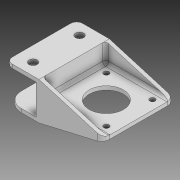
# Autodesk Inventor part: MotorBracket2
Saved by Autodesk Inventor 2020 (Build 240168000, 168)
## iProperties
Created: 2020-10-22
Part Number: MotorBracket2
Material: Generic
Document SubType Name: Modeling
Designer: DDeGo
Density: 1 g/cm^3
Appearance: Default
Author: DDeGo
Autodesk Inventor part; units mm, degrees
ref_plane "YZ Plane" through (0, 0, 0) normal (1, 0, 0) x (0, 1, 0)
ref_plane "XZ Plane" through (0, 0, 0) normal (0, 1, 0) x (-1, 0, 0)
ref_plane "XY Plane" through (0, 0, 0) normal (0, 0, 1) x (1, 0, 0)
sketch "Sketch1" plane through (0, 0, 0) normal (0, 0, 1) x (1, 0, 0)
  line L0 (0, 0) -> (20, 0)
  line L1 (20, 0) -> (20, 2.5) construction
  line L2 (20, 2.5) -> (0, 2.5)
  line L3 (0, 2.5) -> (0, 0)
  line L4 (0, 25.3) -> (20, 25.3)
  line L5 (20, 25.3) -> (20, 22.8) construction
  line L6 (20, 22.8) -> (0, 22.8)
  line L7 (0, 22.8) -> (0, 25.3)
  line L8 (20, 22.8) -> (20, 2.5)
  line L9 (20, 25.3) -> (22, 25.3)
  line L10 (22, 25.3) -> (65.3, 12.5) construction
  line L11 (65.3, 12.5) -> (65.3, 10)
  line L12 (65.3, 10) -> (22, 0) construction
  line L13 (22, 0) -> (20, 0)
  line L14 (22, 25.3) -> (22, 0) construction
  line L15 (22, 25.3) -> (22, 12.5)
  line L16 (65.3, 12.5) -> (22, 12.5)
  line L17 (65.3, 10) -> (22, 10)
  line L18 (22, 10) -> (22, 0)
  dimension "d0" = 2.5
  dimension "d1" = 2.5
  dimension "d2" = 20
  dimension "d3" = 20.3
  dimension "d4" = 2
  dimension "d5" = 43.3
  dimension "d6" = 10
  dimension "d7" = 2.5
  constraints: 38 end point, 6 perpendicular, 4 horizontal, 4 parallel, 4 point on line, 1 collinear, 1 vertical
  measures "d0" distance of L6.end L4.start
  measures "d1" distance of L2.end L0.start
  measures "d2" distance of L0.start L0.end
  measures "d3" distance between parallel lines of L2 L6
  measures "d4" distance between parallel lines of L8 L14
  measures "d5" distance between parallel lines of L11 L14
  measures "d6" distance from line of L2 L10.end
  measures "d7" distance of L10.end L11.end
extrude "Extrusion1" add sketch "Sketch1" along normal mid plane 42.3
sketch "Sketch2" plane through (0, 0, 21.15) normal (0, 0, 1) x (1, 0, 0)
  line L0 (65.3, 10) -> (65.3, 12.5) projected
  line L1 (65.3, 12.5) -> (22, 12.5) construction
  line L2 (22, 12.5) -> (22, 25.3) construction
  line L3 (22, 25.3) -> (0, 25.3) projected
  line L4 (0, 25.3) -> (0, 22.8) projected
  line L5 (0, 22.8) -> (20, 22.8) projected
  line L6 (20, 22.8) -> (20, 2.5) projected
  line L7 (20, 2.5) -> (0, 2.5) projected
  line L8 (0, 2.5) -> (0, 0) projected
  line L9 (0, 0) -> (22, 0) projected
  line L10 (22, 0) -> (22, 10) construction
  line L11 (22, 10) -> (65.3, 10) construction
  line L12 (22, 12.5) -> (22, 25.3) construction
  line L13 (22, 25.3) -> (65.3, 12.5)
  line L14 (65.3, 10) -> (65.3, 12.5) projected
  line L15 (65.3, 10) -> (22, 0)
  constraints: 4 end point
extrude "Extrusion2" add sketch "Sketch2" along normal blind 2.5
mirror "Mirror1" about plane through (0, 0, 0) normal (0, 0, 1) of "Extrusion2"
sketch "Sketch3" plane through (0, 25.3, 23.65) normal (0, 1, 0) x (1, 0, 0)
  line L0 (0, 47.3) -> (22, 47.3) projected
  line L1 (10, 47.3) -> (10, 0) construction
  line L2 (0, 0) -> (20, 0) projected
  circle A0 centre (10, 8) radius 2.75
  circle A1 centre (10, 39.3) radius 2.75
  line L3 (0, 47.3) -> (0, 0) projected
  point P0 (0, 23.65)
  dimension "d12" = 8
  dimension "d13" = 8
  dimension "d14" = 5.5
  dimension "d15" = 10
  constraints: 3 point on line, 2 centre point, 2 end point, 1 equal radius, 1 midpoint, 1 vertical
  measures "d12" distance from line of L0 A1.centre
  measures "d13" distance from line of L2 A0.centre
  measures "d14" diameter of A0
  measures "d15" distance between parallel lines of L3 L1
extrude "Extrusion3" cut sketch "Sketch3" against normal up to surface (2.5 mm away)
sketch "Sketch4" plane through (0, 0, 23.65) normal (0, -1, 0) x (1, 0, 0)
  line L0 (0, -23.65) -> (10, -23.65) construction
  circle A0 centre (10, -23.65) radius 2.75
  dimension "d18" = 5.5
  dimension "d19" = 10
  constraints: 2 end point, 1 centre point, 1 coincident, 1 horizontal
  measures "d18" diameter of A0
  measures "d19" distance of L0.start L0.end
extrude "Extrusion4" cut sketch "Sketch4" against normal up to surface (2.5 mm away)
sketch "Sketch5" plane through (22, 12.5, 21.15) normal (0, 1, 0) x (1, 0, 0)
  line L0 (0, 0) -> (0, -2.5) projected
  line L1 (43.3, 42.3) -> (43.3, 44.8) projected
  line L2 (0, 0) -> (43.3, 42.3) construction
  line L3 (6.15, 5.65) -> (37.15, 5.65) construction
  line L4 (37.15, 5.65) -> (37.15, 36.65) construction
  line L5 (37.15, 36.65) -> (6.15, 36.65) construction
  line L6 (6.15, 36.65) -> (6.15, 5.65) construction
  line L7 (6.15, 5.65) -> (37.15, 36.65) construction
  line L8 (37.15, 5.65) -> (6.15, 36.65) construction
  circle A0 centre (6.15, 36.65) radius 1.75
  circle A1 centre (37.15, 36.65) radius 1.75
  circle A2 centre (37.15, 5.65) radius 1.75
  circle A3 centre (6.15, 5.65) radius 1.75
  circle A4 centre (21.65, 21.15) radius 11.5
  point P0 (-22, 21.15)
  dimension "d22" = 31
  dimension "d23" = 31
  dimension "d24" = 3.5
  dimension "d25" = 23
  constraints: 14 end point, 5 centre point, 5 coincident, 3 equal radius, 3 midpoint, 2 parallel, 1 horizontal, 1 perpendicular
  measures "d22" distance of L3.end L4.end
  measures "d23" distance of L4.end L5.end
  measures "d24" diameter of A1
  measures "d25" diameter of A4
extrude "Extrusion5" cut sketch "Sketch5" against normal through all
fillet "Fillet1" radius 10 2 edges at (0, 1.25, -23.65) (0, 1.25, 23.65)
fillet "Fillet1" radius 4 4 edges at (0, 24.05, -23.65) (0, 24.05, 23.65) (65.3, 11.25, 23.65) (65.3, 11.25, -23.65)
fillet "Fillet1" radius 2 5 edges at (43.65, 12.5, -21.15) (22, 12.5, 0) (43.65, 12.5, 21.15) (22, 18.9, 21.15) (22, 18.9, -21.15)
body "Solid1"
